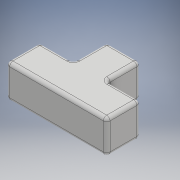
# Autodesk Inventor part: tetris_t
Saved by Autodesk Inventor 2017 (Build 210142000, 142)
## iProperties
Part Number: tetris_t
Material: Všeobecné
Document SubType Name: Modeling
Designer: TM
Density: 1 g/cm^3
Appearance: Výchozí
Author: TM
Autodesk Inventor part; units mm, degrees
ref_plane "YZ Plane" through (0, 0, 0) normal (1, 0, 0) x (0, 1, 0)
ref_plane "XZ Plane" through (0, 0, 0) normal (0, 1, 0) x (-1, 0, 0)
ref_plane "XY Plane" through (0, 0, 0) normal (0, 0, 1) x (1, 0, 0)
sketch "Náčrt1" plane through (0, 0, 0) normal (0, 0, 1) x (1, 0, 0)
  line L0 (0, 0) -> (-0.025, 0) construction
  line L1 (-0.025, 0) -> (-0.025, 0.025) construction
  line L2 (-0.025, 0.025) -> (-0.025, 0.075)
  line L3 (-0.025, 0.075) -> (0.025, 0.075)
  line L4 (0.025, 0.075) -> (0.025, 0.025)
  line L5 (0.025, 0.025) -> (0.075, 0.025)
  line L6 (0.075, 0.025) -> (0.075, -0.025)
  line L7 (0.075, -0.025) -> (-0.075, -0.025)
  line L8 (-0.075, -0.025) -> (-0.075, 0.025)
  line L9 (-0.075, 0.025) -> (-0.025, 0.025)
  dimension "d0" = 0.025
  dimension "d1" = 0.025
  dimension "d2" = 90
  dimension "d3" = 0.05
  dimension "d4" = 0.05
  dimension "d5" = 0.05
  dimension "d6" = 0.05
  dimension "d7" = 0.05
  dimension "d8" = 0.15
  dimension "d9" = 0.05
  constraints: 20 end point, 6 perpendicular, 1 horizontal, 1 point on line, 1 vertical
  measures "d0" distance of L0.start L0.end
  measures "d1" distance of L0.end L1.end
  measures "d2" angle of L0 L1
  measures "d3" distance of L1.end L2.end
  measures "d4" distance of L2.end L3.end
  measures "d5" distance of L3.end L4.end
  measures "d6" distance of L4.end L5.end
  measures "d7" distance of L5.end L6.end
  measures "d8" distance of L6.end L7.end
  measures "d9" distance of L7.end L8.end
extrude "Vysunutí1" add sketch "Náčrt1" along normal mid plane 0.05
fillet "Zaoblení1" radius 0.005 24 edges at (0, -0.025, 0.025) (-0.075, -0.025, 0) (0, -0.025, -0.025) (0.075, -0.025, 0) (0.075, 0, 0.025) (0.075, 0, -0.025) (0.075, 0.025, 0) (-0.075, 0, 0.025) (0.05, 0.025, 0.025) (0.025, 0.05, 0.025) (-0.05, 0.025, 0.025) (-0.025, 0.05, 0.025) (0.05, 0.025, -0.025) (0.025, 0.025, 0) (0.025, 0.05, -0.025) (0.025, 0.075, 0) (0, 0.075, -0.025) (0, 0.075, 0.025) (-0.025, 0.075, 0) (-0.025, 0.05, -0.025) (-0.05, 0.025, -0.025) (-0.075, 0.025, 0) (-0.075, 0, -0.025) (-0.025, 0.025, 0)
